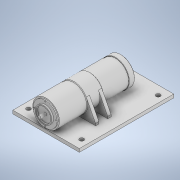
# Autodesk Inventor part: Motor
Saved by Autodesk Inventor 2022.2 (Build 262287000, 287)
## iProperties
Created: 2022-02-10
Part Number: Motor
Material: Genérico
Document SubType Name: Modeling
Designer: USUARIO
Density: 1 g/cm^3
Appearance: Valor por defecto
Author: USUARIO
Autodesk Inventor part; units mm, degrees
ref_plane "YZ Plane" through (0, 0, 0) normal (1, 0, 0) x (0, 1, 0)
sketch "Boceto1" plane through (0, 0, 0) normal (0, 0, 1) x (1, 0, 0)
  circle A0 centre (0, 0) radius 40
  dimension "d0" = 80
  constraints: 1 centre point, 1 coincident
  measures "d0" diameter of A0
extrude "Extrusión1" add sketch "Boceto1" along normal blind 208
sketch "Boceto2" plane through (0, 0, 0) normal (0, 0, -1) x (-1, 0, 0)
  circle A0 centre (0, 0) radius 41.5
  dimension "d3" = 83
  constraints: 1 centre point, 1 coincident
  measures "d3" diameter of A0
extrude "Extrusión2" add sketch "Boceto2" along normal blind 17
fillet "Empalme1" radius 1 2 edges at (41.5, 0, 0) (41.5, 0, -17)
sketch "Boceto3" plane through (0, 0, 208) normal (0, 0, 1) x (1, 0, 0)
  circle A0 centre (0, 0) radius 36
  dimension "d7" = 72
  constraints: 1 centre point, 1 coincident
  measures "d7" diameter of A0
extrude "Extrusión3" add sketch "Boceto3" along normal blind 3
sketch "Boceto4" plane through (0, 0, 211) normal (0, 0, 1) x (1, 0, 0)
  circle A0 centre (0, 0) radius 25
  circle A1 centre (0, 0) radius 22
  dimension "d10" = 50
  dimension "d11" = 44
  constraints: 2 centre point, 2 coincident
  measures "d10" diameter of A0
  measures "d11" diameter of A1
extrude "Extrusión4" add sketch "Boceto4" along normal blind 5
sketch "Boceto5" plane through (0, 0, 211) normal (0, 0, 1) x (1, 0, 0)
  circle A0 centre (0, 0) radius 4.5
  dimension "d14" = 9
  constraints: 1 centre point, 1 coincident
  measures "d14" diameter of A0
extrude "Extrusión5" add sketch "Boceto5" along normal blind 17
sketch "Boceto6" plane through (0, 0, 211) normal (0, 0, 1) x (1, 0, 0)
  circle A0 centre (-32.5, 0) radius 1.5
  circle A1 centre (0, 32.5) radius 1.5
  circle A2 centre (32.5, 0) radius 1.5
  circle A3 centre (0, -32.5) radius 1.5
  point P0 (0, 0)
  dimension "d17" = 3
  dimension "d18" = 3
  dimension "d19" = 3
  dimension "d20" = 3
  dimension "d21" = 65
  dimension "d22" = 65
  dimension "d23" = 32.5
  dimension "d24" = 32.5
  constraints: 4 centre point, 2 horizontal alignment, 2 vertical alignment
  measures "d17" diameter of A0
  measures "d18" diameter of A1
  measures "d19" diameter of A2
  measures "d20" diameter of A3
  measures "d21" distance of A1.centre A3.centre
  measures "d22" distance of A2.centre A0.centre
  measures "d23" distance of A1.centre point (0, 0)
  measures "d24" distance of point (0, 0) A0.centre
extrude "Extrusión6" cut sketch "Boceto6" against normal blind 10
thread "Rosca1" size "M3x0.5" class "6H" standard "ISO Metric profile" length 15
thread "Rosca2" size "M3x0.5" class "6H" standard "ISO Metric profile" length 15
thread "Rosca3" size "M3x0.5" class "6H" standard "ISO Metric profile" length 15
thread "Rosca4" size "M3x0.5" class "6H" standard "ISO Metric profile" length 15
ref_plane "Plano de trabajo1" through (0, 0, 100.75) normal (0, 0, -1) x (-1, 0, 0)
sketch "Boceto7" plane through (0, 0, 100.75) normal (0, 0, -1) x (-1, 0, 0)
  circle A0 centre (0, 0) radius 40 projected
  circle A1 centre (0, 0) radius 41.5
  dimension "d37" = 83
  constraints: 1 centre point, 1 coincident
  measures "d37" diameter of A1
extrude "Extrusión7" add sketch "Boceto7" along normal blind 25 and the other way blind 25.5
fillet "Empalme2" radius 2 2 edges at (41.5, 0, 126.25) (41.5, 0, 75.75)
ref_plane "Plano de trabajo2" through (0, 0, 77.686) normal (0, 0, -1) x (-1, 0, 0)
ref_plane "Plano de trabajo3" through (0, 0, 124.314) normal (0, 0, -1) x (-1, 0, 0)
sketch "Boceto8" plane through (0, 0, 124.314) normal (0, 0, -1) x (-1, 0, 0)
  circle A0 centre (0, 0) radius 41.5 projected
  line L0 (0, -41.5) -> (-65, -41.5)
  line L1 (-65, -41.5) -> (-65, -35.5)
  line L2 (-65, -35.5) -> (-36.8844, 19.0208)
  line L3 (0, -41.5) -> (65, -41.5)
  line L4 (65, -41.5) -> (65, -35.5)
  line L5 (65, -35.5) -> (36.8844, 19.0208)
  dimension "d45" = 6
  dimension "d46" = 65
  dimension "d47" = 65
  dimension "d48" = 6
  constraints: 12 end point, 3 point on circle, 3 tangent, 2 horizontal, 2 perpendicular
  measures "d45" distance of L0.end L1.end
  measures "d46" distance of L0.start L0.end
  measures "d47" distance of L0.start L3.end
  measures "d48" distance of L3.end L4.end
extrude "Extrusión8" add sketch "Boceto8" along normal blind 10 contours A0 L5 L4 L3 | L0 L1 L2 A0
sketch "Boceto9" plane through (0, 0, 77.686) normal (0, 0, -1) x (-1, 0, 0)
  arc A0 (-36.8844, 19.0208) -> (0, -41.5) centre (0, 0) ccw projected
  line L0 (-65, -41.5) -> (0, -41.5) projected
  line L1 (-36.8844, 19.0208) -> (-65, -35.5) projected
  line L2 (-65, -35.5) -> (-65, -41.5) projected
  line L3 (65, -35.5) -> (36.8844, 19.0208) projected
  arc A1 (0, -41.5) -> (36.8844, 19.0208) centre (0, 0) ccw projected
  line L4 (0, -41.5) -> (65, -41.5) projected
  line L5 (65, -41.5) -> (65, -35.5) projected
  point P0 (0, -41.5)
  point P1 (0, -41.5)
  point P2 (0, -41.5)
  point P3 (0, -41.5)
extrude "Extrusión9" add sketch "Boceto9" against normal blind 10
sketch "Boceto10" plane through (0, -41.5, 124.314) normal (0, -1, 0) x (1, 0, 0)
  line L0 (65, 0) -> (0, 0) projected
  line L1 (0, 0) -> (0, -0.0005) projected
  line L2 (0, 0) -> (-65, 0) projected
  line L3 (-65, 0) -> (-65, -10) projected
  line L4 (0, -10) -> (-65, -10) projected
  line L5 (65, -10) -> (0, -10) projected
  line L6 (65, 0) -> (65, -10) projected
  line L7 (65, -46.628) -> (0, -46.628) projected
  line L8 (65, -46.628) -> (65, -36.628) projected
  line L9 (0, -36.628) -> (65, -36.628) projected
  line L10 (-65, -36.628) -> (0, -36.628) projected
  line L11 (-65, -46.628) -> (-65, -36.628) projected
  line L12 (0, -46.628) -> (-65, -46.628) projected
  line L13 (0, -46.628) -> (0, -46.6275) projected
  line L14 (-100, 83.686) -> (100, 83.686)
  line L15 (100, 83.686) -> (100, -200.314)
  line L16 (100, -200.314) -> (-100, -200.314)
  line L17 (-100, -200.314) -> (-100, 83.686)
  line L18 (40, 83.686) -> (-40, 83.686) projected
  circle A0 centre (-80, 56.7285) radius 6.25
  circle A1 centre (80, 56.7285) radius 6.25
  circle A2 centre (-80, -173.3565) radius 6.25
  circle A3 centre (80, -173.3565) radius 6.25
  line L19 (80, -173.3565) -> (-80, -173.3565) construction
  line L20 (-80, 56.7285) -> (-80, -173.3565) construction
  line L21 (-80, 56.7285) -> (80, 56.7285) construction
  line L22 (80, 56.7285) -> (80, -173.3565) construction
  line L23 (0, 83.686) -> (0, -200.314) construction
  line L24 (-100, -58.314) -> (100, -58.314) construction
  point P0 (0, -124.314)
  point P1 (0, 83.686)
  point P2 (0, 56.7285)
  point P3 (0, -58.314)
  point P4 (80, -58.314)
  point P5 (0, -58.314)
  dimension "d53" = 200
  dimension "d54" = 284
  dimension "d55" = 12.5
  dimension "d56" = 12.5
  dimension "d57" = 12.5
  dimension "d58" = 12.5
  dimension "d59" = 160
  dimension "d60" = 160
  dimension "d61" = 230.085
  dimension "d62" = 230.085
  constraints: 20 end point, 9 midpoint, 4 centre point, 3 vertical alignment, 2 parallel, 2 perpendicular, 1 coincident, 1 horizontal, 1 horizontal alignment, 1 vertical
  measures "d53" distance of L15.end L16.end
  measures "d54" distance of L14.end L15.end
  measures "d55" diameter of A0
  measures "d56" diameter of A1
  measures "d57" diameter of A2
  measures "d58" diameter of A3
  measures "d59" distance of L19.start L19.end
  measures "d60" distance of L21.end L20.start
  measures "d61" distance of L19.end L20.start
  measures "d62" distance of L19.start L21.end
extrude "Extrusión10" add sketch "Boceto10" along normal blind 10
